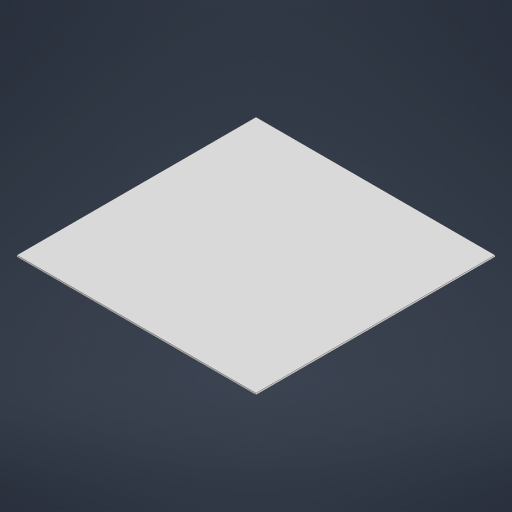
# Autodesk Inventor part: Laminat235x235
Saved by Autodesk Inventor 2023 (Build 270158000, 158)
## iProperties
Created: 2023-04-06
Part Number: Laminat235x235
Material: Generic
Document SubType Name: Modeling
Designer: szykr
Density: 1 g/cm^3
Appearance: Default
Author: szykr
Autodesk Inventor part; units mm, degrees
ref_plane "YZ Plane" through (0, 0, 0) normal (1, 0, 0) x (0, 1, 0)
ref_plane "XZ Plane" through (0, 0, 0) normal (0, 1, 0) x (-1, 0, 0)
ref_plane "XY Plane" through (0, 0, 0) normal (0, 0, 1) x (1, 0, 0)
sketch "Sketch1" plane through (0, 0, 0) normal (0, 1, 0) x (-1, 0, 0)
  line L0 (0, 0) -> (235, 0)
  line L1 (235, 0) -> (235, 235)
  line L2 (235, 235) -> (0, 235)
  line L3 (0, 235) -> (0, 0)
  dimension "d0" = 235
  dimension "d1" = 235
  constraints: 8 end point, 2 parallel, 1 horizontal, 1 perpendicular
  measures "d0" distance of L2.end L1.end
  measures "d1" distance of L1.end L0.end
extrude "Extrusion1" add sketch "Sketch1" along normal blind 1.5
body "Solid1"
